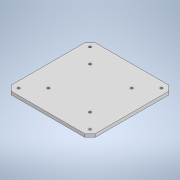
# Autodesk Inventor part: Top Plate
Saved by Autodesk Inventor 2021 (Build 250183000, 183)
## iProperties
Created: 2020-04-12
Part Number: Top Plate
Material: Generic
Document SubType Name: Modeling
Designer: chutsu
Density: 1 g/cm^3
Appearance: Default
Author: chutsu
Autodesk Inventor part; units mm, degrees
ref_plane "YZ Plane" through (0, 0, 0) normal (1, 0, 0) x (0, 1, 0)
ref_plane "XZ Plane" through (0, 0, 0) normal (0, 1, 0) x (-1, 0, 0)
ref_plane "XY Plane" through (0, 0, 0) normal (0, 0, 1) x (1, 0, 0)
sketch "Sketch1" plane through (0, 0, 0) normal (0, 1, 0) x (-1, 0, 0)
  line L0 (40, -40) -> (-40, -40)
  line L1 (-40, -40) -> (-40, 40)
  line L2 (-40, 40) -> (40, 40)
  line L3 (40, 40) -> (40, -40)
  line L4 (40, 0) -> (-40, 0)
  line L5 (0, -40) -> (0, 40)
  point P0 (0, 0)
  dimension "d3" = 80
  dimension "d4" = 80
  constraints: 12 end point, 6 midpoint, 2 parallel, 1 horizontal, 1 perpendicular
  measures "d3" distance between parallel lines of L1 L3
  measures "d4" distance between parallel lines of L2 L0
extrude "Extrusion1" add sketch "Sketch1" along normal blind 3
chamfer "Chamfer1" distance 5 angle 45 4 edges at (-40, 1.5, 40) (40, 1.5, 40) (40, 1.5, -40) (-40, 1.5, -40)
sketch "Sketch3" plane through (0, 3, 0) normal (0, 1, 0) x (1, 0, 0)
  line L0 (35, 40) -> (40, 35) projected
  line L1 (37.5, 37.5) -> (-37.5, -37.5)
  line L2 (-35, -40) -> (-40, -35) projected
  point P0 (0, 0)
  point P1 (19.8223, 19.8223)
  point P2 (33.9645, 33.9645)
  dimension "d12" = 20
  dimension "d13" = 5
  constraints: 2 end point, 2 midpoint, 2 point on line
  measures "d12" distance of point (33.964, 33.964) point (19.822, 19.822)
  measures "d13" distance from line of L0 point (33.964, 33.964)
hole "Hole1" at (19.8223, 3, -19.8223) at (33.9645, 3, -33.9645) direction (0, -1, 0) diameter 2.3 end through all
mirror "Mirror1" about plane through (0, 0, 0) normal (0, 0, 1) of "Hole1"
mirror "Mirror2" about plane through (0, 0, 0) normal (1, 0, 0) of "Hole1", "Mirror1"
body "Solid1"
